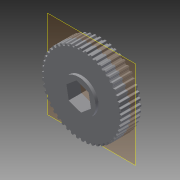
# Autodesk Inventor part: 48T 3mm GT2 - .500 Hex Broach
Saved by Autodesk Inventor 2013 (Build 170138000, 138)
## iProperties
Created: 2013-08-23
Part Number: 48T 3mm GT2 - .500 Hex Broach
Material: Generic
Document SubType Name: Modeling
Designer: grtstudent
Density: 1 g/cm^3
Author: grtstudent
Autodesk Inventor part; units mm, degrees
ref_plane "YZ Plane" through (0, 0, 0) normal (1, 0, 0) x (0, 1, 0)
ref_plane "XZ Plane" through (0, 0, 0) normal (0, 1, 0) x (-1, 0, 0)
ref_plane "XY Plane" through (0, 0, 0) normal (0, 0, 1) x (1, 0, 0)
sketch "Sketch1" plane through (0, 0, 0) normal (0, 0, 1) x (1, 0, 0)
  line L0 (-26.8737, -11.5368) -> (-28.1469, -4.3158)
  line L1 (-28.1469, -4.3158) -> (-22.53, 0.3973)
  line L2 (-22.53, 0.3973) -> (-15.6399, -2.1105)
  line L3 (-15.6399, -2.1105) -> (-14.3666, -9.3314)
  line L4 (-14.3666, -9.3314) -> (-19.9835, -14.0446)
  line L5 (-19.9835, -14.0446) -> (-26.8737, -11.5368)
  arc A0 (-1.0576, 0.1682) -> (-0.8214, 0) centre (-0.8214, 0.25) ccw
  arc A1 (-1.0576, 0.1682) -> (-1.2891, 0.8041) centre (-21.2568, -6.8236) ccw
  arc A2 (-1.2162, 1.0848) -> (-1.2891, 0.8041) centre (-1.0555, 0.8933) ccw
  line L6 (-1.2162, 1.0848) -> (-0.587, 1.6128)
  arc A3 (-0.587, 1.6128) -> (-0.5173, 1.9012) centre (-0.7477, 1.8043) ccw
  arc A4 (-0.5173, 1.9012) -> (-0.8127, 2.5727) centre (-21.2568, -6.8236) ccw
  arc A5 (-0.8127, 2.5727) -> (-1.0725, 2.7162) centre (-1.0399, 2.4683) ccw
  line L7 (-1.0725, 2.7162) -> (-1.8869, 2.609)
  arc A6 (-2.1431, 2.7449) -> (-1.8869, 2.609) centre (-1.9195, 2.8568) ccw
  arc A7 (-2.1431, 2.7449) -> (-2.4555, 3.3451) centre (-21.2568, -6.8236) ccw
  arc A8 (-2.4199, 3.633) -> (-2.4555, 3.3451) centre (-2.2356, 3.4641) ccw
  line L8 (-2.4199, 3.633) -> (-1.865, 4.2385)
  arc A9 (-1.865, 4.2385) -> (-1.8335, 4.5336) centre (-2.0493, 4.4074) ccw
  arc A10 (-1.8335, 4.5336) -> (-2.2141, 5.1608) centre (-21.2568, -6.8236) ccw
  arc A11 (-2.2141, 5.1608) -> (-2.4904, 5.2691) centre (-2.4257, 5.0277) ccw
  line L9 (-2.4904, 5.2691) -> (-3.2838, 5.0566)
  arc A12 (-3.5555, 5.1579) -> (-3.2838, 5.0566) centre (-3.3485, 5.298) ccw
  arc A13 (-3.5555, 5.1579) -> (-3.9436, 5.7122) centre (-21.2568, -6.8236) ccw
  arc A14 (-3.9459, 6.0022) -> (-3.9436, 5.7122) centre (-3.7411, 5.8588) ccw
  line L10 (-3.9459, 6.0022) -> (-3.4748, 6.675)
  arc A15 (-3.4748, 6.675) -> (-3.4821, 6.9717) centre (-3.6796, 6.8184) ccw
  arc A16 (-3.4821, 6.9717) -> (-3.9413, 7.5439) centre (-21.2568, -6.8236) ccw
  arc A17 (-3.9413, 7.5439) -> (-4.2294, 7.6152) centre (-4.1337, 7.3842) ccw
  line L11 (-4.2294, 7.6152) -> (-4.9882, 7.3009)
  arc A18 (-5.2709, 7.3659) -> (-4.9882, 7.3009) centre (-5.0839, 7.5318) ccw
  arc A19 (-5.2709, 7.3659) -> (-5.728, 7.8648) centre (-21.2568, -6.8236) ccw
  arc A20 (-5.7681, 8.152) -> (-5.728, 7.8648) centre (-5.5464, 8.0366) ccw
  line L12 (-5.7681, 8.152) -> (-5.3889, 8.8806)
  arc A21 (-5.3889, 8.8806) -> (-5.4348, 9.1738) centre (-5.6106, 8.996) ccw
  arc A22 (-5.4348, 9.1738) -> (-5.9648, 9.6811) centre (-21.2568, -6.8236) ccw
  arc A23 (-5.9648, 9.6811) -> (-6.2597, 9.7142) centre (-6.1347, 9.4977) ccw
  line L13 (-6.2597, 9.7142) -> (-6.971, 9.3035)
  arc A24 (-7.2597, 9.3311) -> (-6.971, 9.3035) centre (-7.096, 9.52) ccw
  arc A25 (-7.2597, 9.3311) -> (-7.7781, 9.766) centre (-21.2568, -6.8236) ccw
  arc A26 (-7.8554, 10.0455) -> (-7.7781, 9.766) centre (-7.6204, 9.96) ccw
  line L14 (-7.8554, 10.0455) -> (-7.5744, 10.8174)
  arc A27 (-7.5744, 10.8174) -> (-7.6583, 11.1021) centre (-7.8093, 10.9029) ccw
  arc A28 (-7.6583, 11.1021) -> (-8.2499, 11.5359) centre (-21.2568, -6.8236) ccw
  arc A29 (-8.2499, 11.5359) -> (-8.5466, 11.5302) centre (-8.3944, 11.3319) ccw
  line L15 (-8.5466, 11.5302) -> (-9.1982, 11.0302)
  arc A30 (-9.4881, 11.0198) -> (-9.1982, 11.0302) centre (-9.3504, 11.2285) ccw
  arc A31 (-9.4881, 11.0198) -> (-10.0588, 11.3834) centre (-21.2568, -6.8236) ccw
  arc A32 (-10.1719, 11.6505) -> (-10.0588, 11.3834) centre (-9.9278, 11.5964) ccw
  line L16 (-10.1719, 11.6505) -> (-9.9941, 12.4524)
  arc A33 (-9.9941, 12.4524) -> (-10.1144, 12.7237) centre (-10.2382, 12.5065) ccw
  arc A34 (-10.1144, 12.7237) -> (-10.7576, 13.0765) centre (-21.2568, -6.8236) ccw
  arc A35 (-10.7576, 13.0765) -> (-11.051, 13.0322) centre (-10.8742, 12.8554) ccw
  line L17 (-11.051, 13.0322) -> (-11.6318, 12.4514)
  arc A36 (-11.9178, 12.4033) -> (-11.6318, 12.4514) centre (-11.8086, 12.6282) ccw
  arc A37 (-11.9178, 12.4033) -> (-12.5311, 12.6893) centre (-21.2568, -6.8236) ccw
  arc A38 (-12.6781, 12.9393) -> (-12.5311, 12.6893) centre (-12.429, 12.9175) ccw
  line L18 (-12.6781, 12.9393) -> (-12.6065, 13.7575)
  arc A39 (-12.6065, 13.7575) -> (-12.7611, 14.0108) centre (-12.8555, 13.7793) ccw
  arc A40 (-12.7611, 14.0108) -> (-13.4449, 14.2767) centre (-21.2568, -6.8236) ccw
  arc A41 (-13.4449, 14.2767) -> (-13.73, 14.1945) centre (-13.5317, 14.0423) ccw
  line L19 (-13.73, 14.1945) -> (-14.23, 13.5428)
  arc A42 (-14.5073, 13.4578) -> (-14.23, 13.5428) centre (-14.4284, 13.695) ccw
  arc A43 (-14.5073, 13.4578) -> (-15.1527, 13.6613) centre (-21.2568, -6.8236) ccw
  arc A44 (-15.331, 13.89) -> (-15.1527, 13.6613) centre (-15.0813, 13.9009) ccw
  line L20 (-15.331, 13.89) -> (-15.3669, 14.7106)
  arc A45 (-15.3669, 14.7106) -> (-15.5532, 14.9415) centre (-15.6166, 14.6997) ccw
  arc A46 (-15.5532, 14.9415) -> (-16.2658, 15.1159) centre (-21.2568, -6.8236) ccw
  arc A47 (-16.2658, 15.1159) -> (-16.5378, 14.9971) centre (-16.3213, 14.8721) ccw
  line L21 (-16.5378, 14.9971) -> (-16.9485, 14.2857)
  arc A48 (-17.2123, 14.1653) -> (-16.9485, 14.2857) centre (-17.165, 14.4107) ccw
  arc A49 (-17.2123, 14.1653) -> (-17.8787, 14.2828) centre (-21.2568, -6.8236) ccw
  arc A50 (-18.0854, 14.4862) -> (-17.8787, 14.2828) centre (-17.8392, 14.5296) ccw
  line L22 (-18.0854, 14.4862) -> (-18.228, 15.2951)
  arc A51 (-18.228, 15.2951) -> (-18.443, 15.4997) centre (-18.4742, 15.2517) ccw
  arc A52 (-18.443, 15.4997) -> (-19.1722, 15.5796) centre (-21.2568, -6.8236) ccw
  arc A53 (-19.1722, 15.5796) -> (-19.4264, 15.4264) centre (-19.1954, 15.3307) ccw
  line L23 (-19.4264, 15.4264) -> (-19.7407, 14.6675)
  arc A54 (-19.9865, 14.5136) -> (-19.7407, 14.6675) centre (-19.9717, 14.7632) ccw
  arc A55 (-19.9865, 14.5136) -> (-20.6625, 14.5431) centre (-21.2568, -6.8236) ccw
  arc A56 (-20.894, 14.7179) -> (-20.6625, 14.5431) centre (-20.6556, 14.793) ccw
  line L24 (-20.894, 14.7179) -> (-21.141, 15.5012)
  arc A57 (-21.141, 15.5012) -> (-21.3808, 15.676) centre (-21.3794, 15.426) ccw
  arc A58 (-21.3808, 15.676) -> (-22.1143, 15.66) centre (-21.2568, -6.8236) ccw
  arc A59 (-22.1143, 15.66) -> (-22.3462, 15.4749) centre (-22.1047, 15.4102) ccw
  line L25 (-22.3462, 15.4749) -> (-22.5588, 14.6815)
  arc A60 (-22.7824, 14.4969) -> (-22.5588, 14.6815) centre (-22.8003, 14.7462) ccw
  arc A61 (-22.7824, 14.4969) -> (-23.4565, 14.4379) centre (-21.2568, -6.8236) ccw
  arc A62 (-23.7088, 14.5809) -> (-23.4565, 14.4379) centre (-23.4823, 14.6866) ccw
  line L26 (-23.7088, 14.5809) -> (-24.056, 15.3253)
  arc A63 (-24.056, 15.3253) -> (-24.3165, 15.4674) centre (-24.2825, 15.2197) ccw
  arc A64 (-24.3165, 15.4674) -> (-25.0416, 15.3558) centre (-21.2568, -6.8236) ccw
  arc A65 (-25.0416, 15.3558) -> (-25.2474, 15.142) centre (-24.9996, 15.1093) ccw
  line L27 (-25.2474, 15.142) -> (-25.3547, 14.3276)
  arc A66 (-25.5523, 14.1153) -> (-25.3547, 14.3276) centre (-25.6025, 14.3602) ccw
  arc A67 (-25.5523, 14.1153) -> (-26.2129, 13.9689) centre (-21.2568, -6.8236) ccw
  arc A68 (-26.4817, 14.0777) -> (-26.2129, 13.9689) centre (-26.2709, 14.2121) ccw
  line L28 (-26.4817, 14.0777) -> (-26.923, 14.7705)
  arc A69 (-26.923, 14.7705) -> (-27.1999, 14.8773) centre (-27.1339, 14.6362) ccw
  arc A70 (-27.1999, 14.8773) -> (-27.9042, 14.672) centre (-21.2568, -6.8236) ccw
  arc A71 (-27.9042, 14.672) -> (-28.0804, 14.4332) centre (-27.8304, 14.4332) ccw
  line L29 (-28.0804, 14.4332) -> (-28.0804, 13.6118)
  arc A72 (-28.2486, 13.3755) -> (-28.0804, 13.6118) centre (-28.3304, 13.6118) ccw
  arc A73 (-28.2486, 13.3755) -> (-28.8845, 13.1441) centre (-21.2568, -6.8236) ccw
  arc A74 (-29.1652, 13.2169) -> (-28.8845, 13.1441) centre (-28.9737, 13.3776) ccw
  line L30 (-29.1652, 13.2169) -> (-29.6932, 13.8461)
  arc A75 (-29.6932, 13.8461) -> (-29.9816, 13.9159) centre (-29.8847, 13.6855) ccw
  arc A76 (-29.9816, 13.9159) -> (-30.6531, 13.6204) centre (-21.2568, -6.8236) ccw
  arc A77 (-30.6531, 13.6204) -> (-30.7966, 13.3606) centre (-30.5487, 13.3933) ccw
  line L31 (-30.7966, 13.3606) -> (-30.6894, 12.5463)
  arc A78 (-30.8253, 12.2901) -> (-30.6894, 12.5463) centre (-30.9372, 12.5136) ccw
  arc A79 (-30.8253, 12.2901) -> (-31.4255, 11.9776) centre (-21.2568, -6.8236) ccw
  arc A80 (-31.7133, 12.0132) -> (-31.4255, 11.9776) centre (-31.5444, 12.1975) ccw
  line L32 (-31.7133, 12.0132) -> (-32.3189, 12.5681)
  arc A81 (-32.3189, 12.5681) -> (-32.614, 12.5996) centre (-32.4878, 12.3838) ccw
  arc A82 (-32.614, 12.5996) -> (-33.2412, 12.2191) centre (-21.2568, -6.8236) ccw
  arc A83 (-33.2412, 12.2191) -> (-33.3495, 11.9428) centre (-33.108, 12.0075) ccw
  line L33 (-33.3495, 11.9428) -> (-33.1369, 11.1494)
  arc A84 (-33.2383, 10.8776) -> (-33.1369, 11.1494) centre (-33.3784, 11.0847) ccw
  arc A85 (-33.2383, 10.8776) -> (-33.7926, 10.4895) centre (-21.2568, -6.8236) ccw
  arc A86 (-34.0826, 10.4872) -> (-33.7926, 10.4895) centre (-33.9392, 10.692) ccw
  line L34 (-34.0826, 10.4872) -> (-34.7554, 10.9583)
  arc A87 (-34.7554, 10.9583) -> (-35.0521, 10.9511) centre (-34.8988, 10.7536) ccw
  arc A88 (-35.0521, 10.9511) -> (-35.6242, 10.4919) centre (-21.2568, -6.8236) ccw
  arc A89 (-35.6242, 10.4919) -> (-35.6956, 10.2038) centre (-35.4646, 10.2995) ccw
  line L35 (-35.6956, 10.2038) -> (-35.3812, 9.4449)
  arc A90 (-35.4463, 9.1623) -> (-35.3812, 9.4449) centre (-35.6122, 9.3493) ccw
  arc A91 (-35.4463, 9.1623) -> (-35.9451, 8.7051) centre (-21.2568, -6.8236) ccw
  arc A92 (-36.2324, 8.665) -> (-35.9451, 8.7051) centre (-36.1169, 8.8868) ccw
  line L36 (-36.2324, 8.665) -> (-36.961, 9.0443)
  arc A93 (-36.961, 9.0443) -> (-37.2541, 8.9983) centre (-37.0764, 8.8225) ccw
  arc A94 (-37.2541, 8.9983) -> (-37.7615, 8.4684) centre (-21.2568, -6.8236) ccw
  arc A95 (-37.7615, 8.4684) -> (-37.7946, 8.1735) centre (-37.5781, 8.2985) ccw
  line L37 (-37.7946, 8.1735) -> (-37.3839, 7.4621)
  arc A96 (-37.4114, 7.1734) -> (-37.3839, 7.4621) centre (-37.6004, 7.3371) ccw
  arc A97 (-37.4114, 7.1734) -> (-37.8464, 6.6551) centre (-21.2568, -6.8236) ccw
  arc A98 (-38.1259, 6.5778) -> (-37.8464, 6.6551) centre (-38.0404, 6.8127) ccw
  line L38 (-38.1259, 6.5778) -> (-38.8978, 6.8587)
  arc A99 (-38.8978, 6.8587) -> (-39.1825, 6.7749) centre (-38.9833, 6.6238) ccw
  arc A100 (-39.1825, 6.7749) -> (-39.6163, 6.1833) centre (-21.2568, -6.8236) ccw
  arc A101 (-39.6163, 6.1833) -> (-39.6106, 5.8866) centre (-39.4123, 6.0387) ccw
  line L39 (-39.6106, 5.8866) -> (-39.1106, 5.2349)
  arc A102 (-39.1002, 4.9451) -> (-39.1106, 5.2349) centre (-39.3089, 5.0827) ccw
  arc A103 (-39.1002, 4.9451) -> (-39.4638, 4.3744) centre (-21.2568, -6.8236) ccw
  arc A104 (-39.7308, 4.2613) -> (-39.4638, 4.3744) centre (-39.6767, 4.5054) ccw
  line L40 (-39.7308, 4.2613) -> (-40.5328, 4.4391)
  arc A105 (-40.5328, 4.4391) -> (-40.8041, 4.3188) centre (-40.5869, 4.195) ccw
  arc A106 (-40.8041, 4.3188) -> (-41.1569, 3.6756) centre (-21.2568, -6.8236) ccw
  arc A107 (-41.1569, 3.6756) -> (-41.1126, 3.3822) centre (-40.9358, 3.5589) ccw
  line L41 (-41.1126, 3.3822) -> (-40.5318, 2.8014)
  arc A108 (-40.4837, 2.5153) -> (-40.5318, 2.8014) centre (-40.7086, 2.6246) ccw
  arc A109 (-40.4837, 2.5153) -> (-40.7697, 1.9021) centre (-21.2568, -6.8236) ccw
  arc A110 (-41.0197, 1.7551) -> (-40.7697, 1.9021) centre (-40.9979, 2.0041) ccw
  line L42 (-41.0197, 1.7551) -> (-41.8379, 1.8267)
  arc A111 (-41.8379, 1.8267) -> (-42.0912, 1.672) centre (-41.8597, 1.5776) ccw
  arc A112 (-42.0912, 1.672) -> (-42.3571, 0.9883) centre (-21.2568, -6.8236) ccw
  arc A113 (-42.3571, 0.9883) -> (-42.2748, 0.7031) centre (-42.1227, 0.9015) ccw
  line L43 (-42.2748, 0.7031) -> (-41.6232, 0.2031)
  arc A114 (-41.5382, -0.0742) -> (-41.6232, 0.2031) centre (-41.7754, 0.0048) ccw
  arc A115 (-41.5382, -0.0742) -> (-41.7416, -0.7195) centre (-21.2568, -6.8236) ccw
  arc A116 (-41.9703, -0.8979) -> (-41.7416, -0.7195) centre (-41.9812, -0.6481) ccw
  line L44 (-41.9703, -0.8979) -> (-42.7909, -0.9337)
  arc A117 (-42.7909, -0.9337) -> (-43.0219, -1.1201) centre (-42.78, -1.1835) ccw
  arc A118 (-43.0219, -1.1201) -> (-43.1962, -1.8327) centre (-21.2568, -6.8236) ccw
  arc A119 (-43.1962, -1.8327) -> (-43.0775, -2.1047) centre (-42.9525, -1.8882) ccw
  line L45 (-43.0775, -2.1047) -> (-42.3661, -2.5154)
  arc A120 (-42.2456, -2.7792) -> (-42.3661, -2.5154) centre (-42.4911, -2.7319) ccw
  arc A121 (-42.2456, -2.7792) -> (-42.3631, -3.4455) centre (-21.2568, -6.8236) ccw
  arc A122 (-42.5666, -3.6522) -> (-42.3631, -3.4455) centre (-42.61, -3.406) ccw
  line L46 (-42.5666, -3.6522) -> (-43.3755, -3.7949)
  arc A123 (-43.3755, -3.7949) -> (-43.5801, -4.0098) centre (-43.3321, -4.0411) ccw
  arc A124 (-43.5801, -4.0098) -> (-43.66, -4.7391) centre (-21.2568, -6.8236) ccw
  arc A125 (-43.66, -4.7391) -> (-43.5067, -4.9932) centre (-43.4111, -4.7622) ccw
  line L47 (-43.5067, -4.9932) -> (-42.7479, -5.3075)
  arc A126 (-42.594, -5.5534) -> (-42.7479, -5.3075) centre (-42.8435, -5.5385) ccw
  arc A127 (-42.594, -5.5534) -> (-42.6235, -6.2294) centre (-21.2568, -6.8236) ccw
  arc A128 (-42.7982, -6.4609) -> (-42.6235, -6.2294) centre (-42.8734, -6.2224) ccw
  line L48 (-42.7982, -6.4609) -> (-43.5816, -6.7079)
  arc A129 (-43.5816, -6.7079) -> (-43.7564, -6.9477) centre (-43.5064, -6.9463) ccw
  arc A130 (-43.7564, -6.9477) -> (-43.7404, -7.6811) centre (-21.2568, -6.8236) ccw
  arc A131 (-43.7404, -7.6811) -> (-43.5553, -7.9131) centre (-43.4906, -7.6716) ccw
  line L49 (-43.5553, -7.9131) -> (-42.7619, -8.1257)
  arc A132 (-42.5772, -8.3493) -> (-42.7619, -8.1257) centre (-42.8266, -8.3671) ccw
  arc A133 (-42.5772, -8.3493) -> (-42.5183, -9.0234) centre (-21.2568, -6.8236) ccw
  arc A134 (-42.6613, -9.2757) -> (-42.5183, -9.0234) centre (-42.7669, -9.0491) ccw
  line L50 (-42.6613, -9.2757) -> (-43.4057, -9.6228)
  arc A135 (-43.4057, -9.6228) -> (-43.5477, -9.8834) centre (-43.3001, -9.8494) ccw
  arc A136 (-43.5477, -9.8834) -> (-43.4361, -10.6085) centre (-21.2568, -6.8236) ccw
  arc A137 (-43.4361, -10.6085) -> (-43.2223, -10.8143) centre (-43.1897, -10.5664) ccw
  line L51 (-43.2223, -10.8143) -> (-42.408, -10.9215)
  arc A138 (-42.1957, -11.1191) -> (-42.408, -10.9215) centre (-42.4406, -11.1694) ccw
  arc A139 (-42.1957, -11.1191) -> (-42.0493, -11.7797) centre (-21.2568, -6.8236) ccw
  arc A140 (-42.1581, -12.0486) -> (-42.0493, -11.7797) centre (-42.2924, -11.8377) ccw
  line L52 (-42.1581, -12.0486) -> (-42.8509, -12.4899)
  arc A141 (-42.8509, -12.4899) -> (-42.9577, -12.7668) centre (-42.7165, -12.7007) ccw
  arc A142 (-42.9577, -12.7668) -> (-42.7524, -13.4711) centre (-21.2568, -6.8236) ccw
  arc A143 (-42.7524, -13.4711) -> (-42.5135, -13.6472) centre (-42.5135, -13.3972) ccw
  line L53 (-42.5135, -13.6472) -> (-41.6921, -13.6472)
  arc A144 (-41.4559, -13.8155) -> (-41.6921, -13.6472) centre (-41.6921, -13.8972) ccw
  arc A145 (-41.4559, -13.8155) -> (-41.2245, -14.4513) centre (-21.2568, -6.8236) ccw
  arc A146 (-41.2973, -14.732) -> (-41.2245, -14.4513) centre (-41.458, -14.5405) ccw
  line L54 (-41.2973, -14.732) -> (-41.9265, -15.26)
  arc A147 (-41.9265, -15.26) -> (-41.9963, -15.5485) centre (-41.7658, -15.4515) ccw
  arc A148 (-41.9963, -15.5485) -> (-41.7008, -16.22) centre (-21.2568, -6.8236) ccw
  arc A149 (-41.7008, -16.22) -> (-41.441, -16.3634) centre (-41.4736, -16.1156) ccw
  line L55 (-41.441, -16.3634) -> (-40.6267, -16.2562)
  arc A150 (-40.3705, -16.3922) -> (-40.6267, -16.2562) centre (-40.594, -16.5041) ccw
  arc A151 (-40.3705, -16.3922) -> (-40.058, -16.9924) centre (-21.2568, -6.8236) ccw
  arc A152 (-40.0936, -17.2802) -> (-40.058, -16.9924) centre (-40.2779, -17.1113) ccw
  line L56 (-40.0936, -17.2802) -> (-40.6485, -17.8858)
  arc A153 (-40.6485, -17.8858) -> (-40.68, -18.1809) centre (-40.4642, -18.0547) ccw
  arc A154 (-40.68, -18.1809) -> (-40.2994, -18.8081) centre (-21.2568, -6.8236) ccw
  arc A155 (-40.2994, -18.8081) -> (-40.0231, -18.9164) centre (-40.0878, -18.6749) ccw
  line L57 (-40.0231, -18.9164) -> (-39.2297, -18.7038)
  arc A156 (-38.958, -18.8051) -> (-39.2297, -18.7038) centre (-39.165, -18.9453) ccw
  arc A157 (-38.958, -18.8051) -> (-38.5699, -19.3594) centre (-21.2568, -6.8236) ccw
  arc A158 (-38.5676, -19.6494) -> (-38.5699, -19.3594) centre (-38.7724, -19.506) ccw
  line L58 (-38.5676, -19.6494) -> (-39.0387, -20.3223)
  arc A159 (-39.0387, -20.3223) -> (-39.0314, -20.6189) centre (-38.8339, -20.4657) ccw
  arc A160 (-39.0314, -20.6189) -> (-38.5722, -21.1911) centre (-21.2568, -6.8236) ccw
  arc A161 (-38.5722, -21.1911) -> (-38.2842, -21.2624) centre (-38.3798, -21.0315) ccw
  line L59 (-38.2842, -21.2624) -> (-37.5253, -20.9481)
  arc A162 (-37.2427, -21.0131) -> (-37.5253, -20.9481) centre (-37.4296, -21.1791) ccw
  arc A163 (-37.2427, -21.0131) -> (-36.7855, -21.512) centre (-21.2568, -6.8236) ccw
  arc A164 (-36.7454, -21.7992) -> (-36.7855, -21.512) centre (-36.9671, -21.6838) ccw
  line L60 (-36.7454, -21.7992) -> (-37.1247, -22.5278)
  arc A165 (-37.1247, -22.5278) -> (-37.0787, -22.821) centre (-36.9029, -22.6432) ccw
  arc A166 (-37.0787, -22.821) -> (-36.5488, -23.3283) centre (-21.2568, -6.8236) ccw
  arc A167 (-36.5488, -23.3283) -> (-36.2539, -23.3614) centre (-36.3789, -23.1449) ccw
  line L61 (-36.2539, -23.3614) -> (-35.5425, -22.9507)
  arc A168 (-35.2538, -22.9783) -> (-35.5425, -22.9507) centre (-35.4175, -23.1672) ccw
  arc A169 (-35.2538, -22.9783) -> (-34.7355, -23.4132) centre (-21.2568, -6.8236) ccw
  arc A170 (-34.6582, -23.6928) -> (-34.7355, -23.4132) centre (-34.8931, -23.6073) ccw
  line L62 (-34.6582, -23.6928) -> (-34.9391, -24.4646)
  arc A171 (-34.9391, -24.4646) -> (-34.8553, -24.7493) centre (-34.7042, -24.5501) ccw
  arc A172 (-34.8553, -24.7493) -> (-34.2636, -25.1831) centre (-21.2568, -6.8236) ccw
  arc A173 (-34.2636, -25.1831) -> (-33.9669, -25.1775) centre (-34.1191, -24.9791) ccw
  line L63 (-33.9669, -25.1775) -> (-33.3153, -24.6774)
  arc A174 (-33.0254, -24.6671) -> (-33.3153, -24.6774) centre (-33.1631, -24.8758) ccw
  arc A175 (-33.0254, -24.6671) -> (-32.4548, -25.0306) centre (-21.2568, -6.8236) ccw
  arc A176 (-32.3417, -25.2977) -> (-32.4548, -25.0306) centre (-32.5857, -25.2436) ccw
  line L64 (-32.3417, -25.2977) -> (-32.5194, -26.0996)
  arc A177 (-32.5194, -26.0996) -> (-32.3992, -26.3709) centre (-32.2754, -26.1537) ccw
  arc A178 (-32.3992, -26.3709) -> (-31.756, -26.7238) centre (-21.2568, -6.8236) ccw
  arc A179 (-31.756, -26.7238) -> (-31.4625, -26.6794) centre (-31.6393, -26.5027) ccw
  line L65 (-31.4625, -26.6794) -> (-30.8817, -26.0986)
  arc A180 (-30.5957, -26.0505) -> (-30.8817, -26.0986) centre (-30.705, -26.2754) ccw
  arc A181 (-30.5957, -26.0505) -> (-29.9825, -26.3365) centre (-21.2568, -6.8236) ccw
  arc A182 (-29.8355, -26.5865) -> (-29.9825, -26.3365) centre (-30.0845, -26.5647) ccw
  line L66 (-29.8355, -26.5865) -> (-29.9071, -27.4048)
  arc A183 (-29.9071, -27.4048) -> (-29.7524, -27.6581) centre (-29.658, -27.4266) ccw
  arc A184 (-29.7524, -27.6581) -> (-29.0687, -27.924) centre (-21.2568, -6.8236) ccw
  arc A185 (-29.0687, -27.924) -> (-28.7835, -27.8417) centre (-28.9819, -27.6895) ccw
  line L67 (-28.7835, -27.8417) -> (-28.2835, -27.19)
  arc A186 (-28.0062, -27.105) -> (-28.2835, -27.19) centre (-28.0852, -27.3422) ccw
  arc A187 (-28.0062, -27.105) -> (-27.3609, -27.3085) centre (-21.2568, -6.8236) ccw
  arc A188 (-27.1825, -27.5372) -> (-27.3609, -27.3085) centre (-27.4323, -27.5481) ccw
  line L68 (-27.1825, -27.5372) -> (-27.1467, -28.3578)
  arc A189 (-27.1467, -28.3578) -> (-26.9603, -28.5887) centre (-26.8969, -28.3469) ccw
  arc A190 (-26.9603, -28.5887) -> (-26.2477, -28.7631) centre (-21.2568, -6.8236) ccw
  arc A191 (-26.2477, -28.7631) -> (-25.9757, -28.6443) centre (-26.1922, -28.5193) ccw
  line L69 (-25.9757, -28.6443) -> (-25.565, -27.933)
  arc A192 (-25.3012, -27.8125) -> (-25.565, -27.933) centre (-25.3485, -28.058) ccw
  arc A193 (-25.3012, -27.8125) -> (-24.6348, -27.93) centre (-21.2568, -6.8236) ccw
  arc A194 (-24.4281, -28.1334) -> (-24.6348, -27.93) centre (-24.6744, -28.1769) ccw
  line L70 (-24.4281, -28.1334) -> (-24.2855, -28.9424)
  arc A195 (-24.2855, -28.9424) -> (-24.0706, -29.147) centre (-24.0393, -28.8989) ccw
  arc A196 (-24.0706, -29.147) -> (-23.3413, -29.2268) centre (-21.2568, -6.8236) ccw
  arc A197 (-23.3413, -29.2268) -> (-23.0872, -29.0736) centre (-23.3181, -28.9779) ccw
  line L71 (-23.0872, -29.0736) -> (-22.7728, -28.3147)
  arc A198 (-22.527, -28.1608) -> (-22.7728, -28.3147) centre (-22.5419, -28.4104) ccw
  arc A199 (-22.527, -28.1608) -> (-21.851, -28.1904) centre (-21.2568, -6.8236) ccw
  arc A200 (-21.6195, -28.3651) -> (-21.851, -28.1904) centre (-21.858, -28.4403) ccw
  line L72 (-21.6195, -28.3651) -> (-21.3725, -29.1485)
  arc A201 (-21.3725, -29.1485) -> (-21.1327, -29.3233) centre (-21.1341, -29.0733) ccw
  arc A202 (-21.1327, -29.3233) -> (-20.3993, -29.3073) centre (-21.2568, -6.8236) ccw
  arc A203 (-20.3993, -29.3073) -> (-20.1673, -29.1222) centre (-20.4088, -29.0575) ccw
  line L73 (-20.1673, -29.1222) -> (-19.9547, -28.3288)
  arc A204 (-19.7311, -28.1441) -> (-19.9547, -28.3288) centre (-19.7132, -28.3935) ccw
  arc A205 (-19.7311, -28.1441) -> (-19.057, -28.0851) centre (-21.2568, -6.8236) ccw
  arc A206 (-18.8047, -28.2281) -> (-19.057, -28.0851) centre (-19.0313, -28.3338) ccw
  line L74 (-18.8047, -28.2281) -> (-18.4576, -28.9726)
  arc A207 (-18.4576, -28.9726) -> (-18.197, -29.1146) centre (-18.231, -28.8669) ccw
  arc A208 (-18.197, -29.1146) -> (-17.4719, -29.003) centre (-21.2568, -6.8236) ccw
  arc A209 (-17.4719, -29.003) -> (-17.2661, -28.7892) centre (-17.514, -28.7566) ccw
  line L75 (-17.2661, -28.7892) -> (-17.1589, -27.9748)
  arc A210 (-16.9613, -27.7626) -> (-17.1589, -27.9748) centre (-16.911, -28.0075) ccw
  arc A211 (-16.9613, -27.7626) -> (-16.3006, -27.6161) centre (-21.2568, -6.8236) ccw
  arc A212 (-16.0318, -27.725) -> (-16.3006, -27.6161) centre (-16.2427, -27.8593) ccw
  line L76 (-16.0318, -27.725) -> (-15.5905, -28.4177)
  arc A213 (-15.5905, -28.4177) -> (-15.3136, -28.5245) centre (-15.3796, -28.2834) ccw
  arc A214 (-15.3136, -28.5245) -> (-14.6093, -28.3192) centre (-21.2568, -6.8236) ccw
  arc A215 (-14.6093, -28.3192) -> (-14.4332, -28.0804) centre (-14.6832, -28.0804) ccw
  line L77 (-14.4332, -28.0804) -> (-14.4332, -27.259)
  arc A216 (-14.2649, -27.0227) -> (-14.4332, -27.259) centre (-14.1832, -27.259) ccw
  arc A217 (-14.2649, -27.0227) -> (-13.6291, -26.7913) centre (-21.2568, -6.8236) ccw
  arc A218 (-13.3484, -26.8642) -> (-13.6291, -26.7913) centre (-13.5399, -27.0249) ccw
  line L78 (-13.3484, -26.8642) -> (-12.8204, -27.4934)
  arc A219 (-12.8204, -27.4934) -> (-12.5319, -27.5631) centre (-12.6289, -27.3327) ccw
  arc A220 (-12.5319, -27.5631) -> (-11.8604, -27.2677) centre (-21.2568, -6.8236) ccw
  arc A221 (-11.8604, -27.2677) -> (-11.717, -27.0079) centre (-11.9648, -27.0405) ccw
  line L79 (-11.717, -27.0079) -> (-11.8242, -26.1935)
  arc A222 (-11.6882, -25.9373) -> (-11.8242, -26.1935) centre (-11.5763, -26.1609) ccw
  arc A223 (-11.6882, -25.9373) -> (-11.088, -25.6249) centre (-21.2568, -6.8236) ccw
  arc A224 (-10.8002, -25.6605) -> (-11.088, -25.6249) centre (-10.9691, -25.8448) ccw
  line L80 (-10.8002, -25.6605) -> (-10.1946, -26.2154)
  arc A225 (-10.1946, -26.2154) -> (-9.8995, -26.2469) centre (-10.0257, -26.0311) ccw
  arc A226 (-9.8995, -26.2469) -> (-9.2723, -25.8663) centre (-21.2568, -6.8236) ccw
  arc A227 (-9.2723, -25.8663) -> (-9.164, -25.59) centre (-9.4055, -25.6547) ccw
  line L81 (-9.164, -25.59) -> (-9.3766, -24.7966)
  arc A228 (-9.2752, -24.5249) -> (-9.3766, -24.7966) centre (-9.1351, -24.7319) ccw
  arc A229 (-9.2752, -24.5249) -> (-8.721, -24.1367) centre (-21.2568, -6.8236) ccw
  arc A230 (-8.431, -24.1344) -> (-8.721, -24.1367) centre (-8.5743, -24.3392) ccw
  line L82 (-8.431, -24.1344) -> (-7.7581, -24.6056)
  arc A231 (-7.7581, -24.6056) -> (-7.4614, -24.5983) centre (-7.6147, -24.4008) ccw
  arc A232 (-7.4614, -24.5983) -> (-6.8893, -24.1391) centre (-21.2568, -6.8236) ccw
  arc A233 (-6.8893, -24.1391) -> (-6.818, -23.851) centre (-7.0489, -23.9467) ccw
  line L83 (-6.818, -23.851) -> (-7.1323, -23.0922)
  arc A234 (-7.0673, -22.8095) -> (-7.1323, -23.0922) centre (-6.9013, -22.9965) ccw
  arc A235 (-7.0673, -22.8095) -> (-6.5684, -22.3524) centre (-21.2568, -6.8236) ccw
  arc A236 (-6.2812, -22.3122) -> (-6.5684, -22.3524) centre (-6.3966, -22.534) ccw
  line L84 (-6.2812, -22.3122) -> (-5.5526, -22.6915)
  arc A237 (-5.5526, -22.6915) -> (-5.2594, -22.6456) centre (-5.4371, -22.4698) ccw
  arc A238 (-5.2594, -22.6456) -> (-4.7521, -22.1156) centre (-21.2568, -6.8236) ccw
  arc A239 (-4.7521, -22.1156) -> (-4.719, -21.8207) centre (-4.9355, -21.9457) ccw
  line L85 (-4.719, -21.8207) -> (-5.1297, -21.1094)
  arc A240 (-5.1021, -20.8207) -> (-5.1297, -21.1094) centre (-4.9131, -20.9844) ccw
  arc A241 (-5.1021, -20.8207) -> (-4.6671, -20.3023) centre (-21.2568, -6.8236) ccw
  arc A242 (-4.3876, -20.225) -> (-4.6671, -20.3023) centre (-4.4731, -20.4599) ccw
  line L86 (-4.3876, -20.225) -> (-3.6158, -20.506)
  arc A243 (-3.6158, -20.506) -> (-3.3311, -20.4221) centre (-3.5302, -20.271) ccw
  arc A244 (-3.3311, -20.4221) -> (-2.8973, -19.8305) centre (-21.2568, -6.8236) ccw
  arc A245 (-2.8973, -19.8305) -> (-2.9029, -19.5338) centre (-3.1013, -19.686) ccw
  line L87 (-2.9029, -19.5338) -> (-3.403, -18.8821)
  arc A246 (-3.4133, -18.5923) -> (-3.403, -18.8821) centre (-3.2046, -18.7299) ccw
  arc A247 (-3.4133, -18.5923) -> (-3.0497, -18.0216) centre (-21.2568, -6.8236) ccw
  arc A248 (-2.7827, -17.9085) -> (-3.0497, -18.0216) centre (-2.8368, -18.1526) ccw
  line L88 (-2.7827, -17.9085) -> (-1.9808, -18.0863)
  arc A249 (-1.9808, -18.0863) -> (-1.7095, -17.966) centre (-1.9267, -17.8422) ccw
  arc A250 (-1.7095, -17.966) -> (-1.3566, -17.3228) centre (-21.2568, -6.8236) ccw
  arc A251 (-1.3566, -17.3228) -> (-1.4009, -17.0294) centre (-1.5777, -17.2062) ccw
  line L89 (-1.4009, -17.0294) -> (-1.9817, -16.4486)
  arc A252 (-2.0298, -16.1626) -> (-1.9817, -16.4486) centre (-1.805, -16.2718) ccw
  arc A253 (-2.0298, -16.1626) -> (-1.7439, -15.5493) centre (-21.2568, -6.8236) ccw
  arc A254 (-1.4939, -15.4023) -> (-1.7439, -15.5493) centre (-1.5157, -15.6514) ccw
  line L90 (-1.4939, -15.4023) -> (-0.6756, -15.4739)
  arc A255 (-0.6756, -15.4739) -> (-0.4223, -15.3193) centre (-0.6538, -15.2249) ccw
  arc A256 (-0.4223, -15.3193) -> (-0.1564, -14.6355) centre (-21.2568, -6.8236) ccw
  arc A257 (-0.1564, -14.6355) -> (-0.2387, -14.3504) centre (-0.3909, -14.5487) ccw
  line L91 (-0.2387, -14.3504) -> (-0.8903, -13.8503)
  arc A258 (-0.9754, -13.5731) -> (-0.8903, -13.8503) centre (-0.7381, -13.652) ccw
  arc A259 (-0.9754, -13.5731) -> (-0.7719, -12.9277) centre (-21.2568, -6.8236) ccw
  arc A260 (-0.5432, -12.7494) -> (-0.7719, -12.9277) centre (-0.5323, -12.9991) ccw
  line L92 (-0.5432, -12.7494) -> (0.2774, -12.7135)
  arc A261 (0.2774, -12.7135) -> (0.5083, -12.5271) centre (0.2665, -12.4638) ccw
  arc A262 (0.5083, -12.5271) -> (0.6827, -11.8145) centre (-21.2568, -6.8236) ccw
  arc A263 (0.6827, -11.8145) -> (0.5639, -11.5426) centre (0.4389, -11.7591) ccw
  line L93 (0.5639, -11.5426) -> (-0.1474, -11.1319)
  arc A264 (-0.2679, -10.8681) -> (-0.1474, -11.1319) centre (-0.0224, -10.9154) ccw
  arc A265 (-0.2679, -10.8681) -> (-0.1504, -10.2017) centre (-21.2568, -6.8236) ccw
  arc A266 (0.0531, -9.995) -> (-0.1504, -10.2017) centre (0.0965, -10.2412) ccw
  line L94 (0.0531, -9.995) -> (0.862, -9.8524)
  arc A267 (0.862, -9.8524) -> (1.0666, -9.6374) centre (0.8186, -9.6062) ccw
  arc A268 (1.0666, -9.6374) -> (1.1465, -8.9082) centre (-21.2568, -6.8236) ccw
  arc A269 (1.1465, -8.9082) -> (0.9932, -8.654) centre (0.8975, -8.885) ccw
  line L95 (0.9932, -8.654) -> (0.2343, -8.3397)
  arc A270 (0.0805, -8.0939) -> (0.2343, -8.3397) centre (0.33, -8.1087) ccw
  arc A271 (0.0805, -8.0939) -> (0.11, -7.4179) centre (-21.2568, -6.8236) ccw
  arc A272 (0.2847, -7.1864) -> (0.11, -7.4179) centre (0.3599, -7.4248) ccw
  line L96 (0.2847, -7.1864) -> (1.0681, -6.9394)
  arc A273 (1.0681, -6.9394) -> (1.2429, -6.6996) centre (0.9929, -6.701) ccw
  arc A274 (1.2429, -6.6996) -> (1.2269, -5.9661) centre (-21.2568, -6.8236) ccw
  arc A275 (1.2269, -5.9661) -> (1.0418, -5.7342) centre (0.9771, -5.9756) ccw
  line L97 (1.0418, -5.7342) -> (0.2484, -5.5216)
  arc A276 (0.0637, -5.2979) -> (0.2484, -5.5216) centre (0.3131, -5.2801) ccw
  arc A277 (0.0637, -5.2979) -> (0.0047, -4.6239) centre (-21.2568, -6.8236) ccw
  arc A278 (0.1478, -4.3715) -> (0.0047, -4.6239) centre (0.2534, -4.5981) ccw
  line L98 (0.1478, -4.3715) -> (0.8922, -4.0244)
  arc A279 (0.8922, -4.0244) -> (1.0342, -3.7638) centre (0.7865, -3.7978) ccw
  arc A280 (1.0342, -3.7638) -> (0.9226, -3.0387) centre (-21.2568, -6.8236) ccw
  arc A281 (0.9226, -3.0387) -> (0.7088, -2.8329) centre (0.6762, -3.0808) ccw
  line L99 (0.7088, -2.8329) -> (-0.1056, -2.7257)
  arc A282 (-0.3178, -2.5281) -> (-0.1056, -2.7257) centre (-0.0729, -2.4779) ccw
  arc A283 (-0.3178, -2.5281) -> (-0.4643, -1.8675) centre (-21.2568, -6.8236) ccw
  arc A284 (-0.3554, -1.5987) -> (-0.4643, -1.8675) centre (-0.2211, -1.8095) ccw
  line L100 (-0.3554, -1.5987) -> (0.3373, -1.1573)
  arc A285 (0.3373, -1.1573) -> (0.4441, -0.8805) centre (0.203, -0.9465) ccw
  arc A286 (0.4441, -0.8805) -> (0.2388, -0.1761) centre (-21.2568, -6.8236) ccw
  arc A287 (0.2388, -0.1761) -> (0, 0) centre (0, -0.25) ccw
  line L101 (0, 0) -> (-0.8214, 0)
  point P0 (0, 0)
  constraints: 576 point on circle, 288 centre point, 204 end point, 2 horizontal, 2 vertical, 1065 other
extrude "Extrusion1" add sketch "Sketch1" along normal blind 11.1125
sketch "Sketch2" plane through (0, 0, 11.1125) normal (0, 0, 1) x (1, 0, 0)
  line L0 (-22.53, 0.3973) -> (-15.6399, -2.1105) projected
  line L1 (-15.6399, -2.1105) -> (-14.3666, -9.3314) projected
  line L2 (-14.3666, -9.3314) -> (-19.9835, -14.0446) projected
  line L3 (-19.9835, -14.0446) -> (-26.8737, -11.5368) projected
  line L4 (-26.8737, -11.5368) -> (-28.1469, -4.3158) projected
  line L5 (-28.1469, -4.3158) -> (-22.53, 0.3973) projected
  arc A0 (0.4441, -0.8805) -> (0.2388, -0.1761) centre (-21.2568, -6.8236) ccw projected
  circle A1 centre (-21.2568, -6.8236) radius 9.525
  dimension "d2" = 19.05
  constraints: 1 centre point, 1 coincident
  measures "d2" diameter of A1
extrude "Extrusion2" add sketch "Sketch2" along normal blind 1.5875
ref_plane "Work Plane1" through (0, 0, 5.5563) normal (0, 0, 1) x (1, 0, 0)
body "Solid1"
